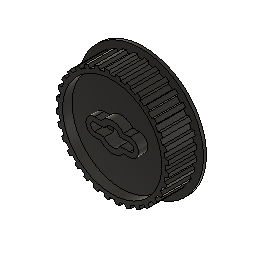
ENGRENAGEM_MEDIA Modificada v1 (Autodesk Fusion 360 design; units mm, degrees)
Autodesk Fusion 360 part; units mm, degrees
note: some values were not read from the file. Set by a fixed rule: which sketch regions a step uses.
sketch "Esboço1" plane through (0, 0, 0) normal (0, 1, 0) x (1, 0, 0)
  circle A0 centre (0, 0) radius 24.25
  line L0 (-0.0462, -30) -> (-0.0462, 30) construction
  circle A1 centre (0, 0) radius 4
  circle A2 centre (0, 0) radius 6.5
  line L1 (0, 0) -> (9.8, 0) construction
  line L2 (0, 0) -> (-9.8, 0) construction
  line L3 (-8, -1.8) -> (8, -1.8)
  arc A3 (8, -1.8) -> (8, 1.8) centre (8, 0) ccw
  line L4 (8, 1.8) -> (-8, 1.8)
  arc A4 (-8, 1.8) -> (-8, -1.8) centre (-8, 0) ccw
  line L5 (-8, 0) -> (8, 0) construction
  line L6 (8, 4) -> (-8, 4)
  arc A5 (-8, 4) -> (-8, -4) centre (-8, 0) ccw
  line L7 (-8, -4) -> (8, -4)
  arc A6 (8, -4) -> (8, 4) centre (8, 0) ccw
  line L8 (8, 0) -> (-8, 0) construction
  circle A7 centre (0, 0) radius 22.561
  circle A8 centre (0, 0) radius 25.6
  line L9 (1.1957, -24.2693) -> (1.7958, -25.976)
  line L10 (-1.0097, -24.2452) -> (1.1957, -24.2693)
  line L11 (1.7958, -25.976) -> (-1.647, -25.9383)
  line L12 (-1.647, -25.9383) -> (-1.0097, -24.2452)
  circle A9 centre (0, 0) radius 25.7968
  line L13 (3.7397, -23.9763) -> (5.9074, -23.5697)
  line L14 (6.829, -25.1265) -> (3.445, -25.7612)
  line L15 (3.445, -25.7612) -> (3.7397, -23.9763)
  line L16 (5.9074, -23.5697) -> (6.829, -25.1265)
  line L17 (8.3454, -22.786) -> (10.3921, -21.9643)
  line L18 (11.5997, -23.3114) -> (8.4045, -24.5941)
  line L19 (8.4045, -24.5941) -> (8.3454, -22.786)
  line L20 (10.3921, -21.9643) -> (11.5997, -23.3114)
  line L21 (12.6304, -20.7201) -> (14.4775, -19.5149)
  line L22 (15.9246, -20.6005) -> (13.0411, -22.4819)
  line L23 (13.0411, -22.4819) -> (12.6304, -20.7201)
  line L24 (14.4775, -19.5149) -> (15.9246, -20.6005)
  line L25 (16.43, -17.8579) -> (18.0065, -16.3155)
  line L26 (19.6376, -17.098) -> (17.1766, -19.5057)
  line L27 (17.1766, -19.5057) -> (16.43, -17.8579)
  line L28 (18.0065, -16.3155) -> (19.6376, -17.098)
  line L29 (19.5982, -14.3094) -> (20.8435, -12.4891)
  line L30 (22.5959, -12.9383) -> (20.6519, -15.78)
  line L31 (20.6519, -15.78) -> (19.5982, -14.3094)
  line L32 (20.8435, -12.4891) -> (22.5959, -12.9383)
  line L33 (22.0132, -10.211) -> (22.8795, -8.1828)
  line L34 (24.6859, -8.2815) -> (23.3336, -11.4478)
  line L35 (23.3336, -11.4478) -> (22.0132, -10.211)
  line L36 (22.8795, -8.1828) -> (24.6859, -8.2815)
  line L37 (23.5823, -5.7203) -> (24.0362, -3.562)
  line L38 (25.8272, -3.3064) -> (25.1186, -6.6756)
  line L39 (25.1186, -6.6756) -> (23.5823, -5.7203)
  line L40 (24.0362, -3.562) -> (25.8272, -3.3064)
  line L41 (24.2452, -1.0097) -> (24.2693, 1.1957)
  line L42 (25.976, 1.7958) -> (25.9383, -1.647)
  line L43 (25.9383, -1.647) -> (24.2452, -1.0097)
  line L44 (24.2693, 1.1957) -> (25.976, 1.7958)
  line L45 (23.9763, 3.7397) -> (23.5697, 5.9074)
  line L46 (25.1265, 6.829) -> (25.7612, 3.445)
  line L47 (25.7612, 3.445) -> (23.9763, 3.7397)
  line L48 (23.5697, 5.9074) -> (25.1265, 6.829)
  line L49 (22.786, 8.3454) -> (21.9643, 10.3921)
  line L50 (23.3114, 11.5997) -> (24.5941, 8.4045)
  line L51 (24.5941, 8.4045) -> (22.786, 8.3454)
  line L52 (21.9643, 10.3921) -> (23.3114, 11.5997)
  line L53 (20.7201, 12.6304) -> (19.5149, 14.4775)
  line L54 (20.6005, 15.9246) -> (22.4819, 13.0411)
  line L55 (22.4819, 13.0411) -> (20.7201, 12.6304)
  line L56 (19.5149, 14.4775) -> (20.6005, 15.9246)
  line L57 (17.8579, 16.43) -> (16.3155, 18.0065)
  line L58 (17.098, 19.6376) -> (19.5057, 17.1766)
  line L59 (19.5057, 17.1766) -> (17.8579, 16.43)
  line L60 (16.3155, 18.0065) -> (17.098, 19.6376)
  line L61 (14.3094, 19.5982) -> (12.4891, 20.8435)
  line L62 (12.9383, 22.5959) -> (15.78, 20.6519)
  line L63 (15.78, 20.6519) -> (14.3094, 19.5982)
  line L64 (12.4891, 20.8435) -> (12.9383, 22.5959)
  line L65 (10.211, 22.0132) -> (8.1828, 22.8795)
  line L66 (8.2815, 24.6859) -> (11.4478, 23.3336)
  line L67 (11.4478, 23.3336) -> (10.211, 22.0132)
  line L68 (8.1828, 22.8795) -> (8.2815, 24.6859)
  line L69 (5.7203, 23.5823) -> (3.562, 24.0362)
  line L70 (3.3064, 25.8272) -> (6.6756, 25.1186)
  line L71 (6.6756, 25.1186) -> (5.7203, 23.5823)
  line L72 (3.562, 24.0362) -> (3.3064, 25.8272)
  line L73 (1.0097, 24.2452) -> (-1.1957, 24.2693)
  line L74 (-1.7958, 25.976) -> (1.647, 25.9383)
  line L75 (1.647, 25.9383) -> (1.0097, 24.2452)
  line L76 (-1.1957, 24.2693) -> (-1.7958, 25.976)
  line L77 (-3.7397, 23.9763) -> (-5.9074, 23.5697)
  line L78 (-6.829, 25.1265) -> (-3.445, 25.7612)
  line L79 (-3.445, 25.7612) -> (-3.7397, 23.9763)
  line L80 (-5.9074, 23.5697) -> (-6.829, 25.1265)
  line L81 (-8.3454, 22.786) -> (-10.3921, 21.9643)
  line L82 (-11.5997, 23.3114) -> (-8.4045, 24.5941)
  line L83 (-8.4045, 24.5941) -> (-8.3454, 22.786)
  line L84 (-10.3921, 21.9643) -> (-11.5997, 23.3114)
  line L85 (-12.6304, 20.7201) -> (-14.4775, 19.5149)
  line L86 (-15.9246, 20.6005) -> (-13.0411, 22.4819)
  line L87 (-13.0411, 22.4819) -> (-12.6304, 20.7201)
  line L88 (-14.4775, 19.5149) -> (-15.9246, 20.6005)
  line L89 (-16.43, 17.8579) -> (-18.0065, 16.3155)
  line L90 (-19.6376, 17.098) -> (-17.1766, 19.5057)
  line L91 (-17.1766, 19.5057) -> (-16.43, 17.8579)
  line L92 (-18.0065, 16.3155) -> (-19.6376, 17.098)
  line L93 (-19.5982, 14.3094) -> (-20.8435, 12.4891)
  line L94 (-22.5959, 12.9383) -> (-20.6519, 15.78)
  line L95 (-20.6519, 15.78) -> (-19.5982, 14.3094)
  line L96 (-20.8435, 12.4891) -> (-22.5959, 12.9383)
  line L97 (-22.0132, 10.211) -> (-22.8795, 8.1828)
  line L98 (-24.6859, 8.2815) -> (-23.3336, 11.4478)
  line L99 (-23.3336, 11.4478) -> (-22.0132, 10.211)
  line L100 (-22.8795, 8.1828) -> (-24.6859, 8.2815)
  line L101 (-23.5823, 5.7203) -> (-24.0362, 3.562)
  line L102 (-25.8272, 3.3064) -> (-25.1186, 6.6756)
  line L103 (-25.1186, 6.6756) -> (-23.5823, 5.7203)
  line L104 (-24.0362, 3.562) -> (-25.8272, 3.3064)
  line L105 (-24.2452, 1.0097) -> (-24.2693, -1.1957)
  line L106 (-25.976, -1.7958) -> (-25.9383, 1.647)
  line L107 (-25.9383, 1.647) -> (-24.2452, 1.0097)
  line L108 (-24.2693, -1.1957) -> (-25.976, -1.7958)
  line L109 (-23.9763, -3.7397) -> (-23.5697, -5.9074)
  line L110 (-25.1265, -6.829) -> (-25.7612, -3.445)
  line L111 (-25.7612, -3.445) -> (-23.9763, -3.7397)
  line L112 (-23.5697, -5.9074) -> (-25.1265, -6.829)
  line L113 (-22.786, -8.3454) -> (-21.9643, -10.3921)
  line L114 (-23.3114, -11.5997) -> (-24.5941, -8.4045)
  line L115 (-24.5941, -8.4045) -> (-22.786, -8.3454)
  line L116 (-21.9643, -10.3921) -> (-23.3114, -11.5997)
  line L117 (-20.7201, -12.6304) -> (-19.5149, -14.4775)
  line L118 (-20.6005, -15.9246) -> (-22.4819, -13.0411)
  line L119 (-22.4819, -13.0411) -> (-20.7201, -12.6304)
  line L120 (-19.5149, -14.4775) -> (-20.6005, -15.9246)
  line L121 (-17.8579, -16.43) -> (-16.3155, -18.0065)
  line L122 (-17.098, -19.6376) -> (-19.5057, -17.1766)
  line L123 (-19.5057, -17.1766) -> (-17.8579, -16.43)
  line L124 (-16.3155, -18.0065) -> (-17.098, -19.6376)
  line L125 (-14.3094, -19.5982) -> (-12.4891, -20.8435)
  line L126 (-12.9383, -22.5959) -> (-15.78, -20.6519)
  line L127 (-15.78, -20.6519) -> (-14.3094, -19.5982)
  line L128 (-12.4891, -20.8435) -> (-12.9383, -22.5959)
  line L129 (-10.211, -22.0132) -> (-8.1828, -22.8795)
  line L130 (-8.2815, -24.6859) -> (-11.4478, -23.3336)
  line L131 (-11.4478, -23.3336) -> (-10.211, -22.0132)
  line L132 (-8.1828, -22.8795) -> (-8.2815, -24.6859)
  line L133 (-5.7203, -23.5823) -> (-3.562, -24.0362)
  line L134 (-3.3064, -25.8272) -> (-6.6756, -25.1186)
  line L135 (-6.6756, -25.1186) -> (-5.7203, -23.5823)
  line L136 (-3.562, -24.0362) -> (-3.3064, -25.8272)
  dimension "d2" = 48.5
  dimension "d7" = 8
  dimension "d8" = 13
  dimension "d10" = 9.8
  dimension "d11" = 9.8
  dimension "d12" = 4
  dimension "d19" = 45.1221
  dimension "d27" = 1.8
  dimension "d65" = 51.2
  dimension "d111" = 70
  dimension "d112" = 70
  dimension "d113" = 2.2055
  dimension "d114" = 3.443
  dimension "d116" = 51.5937
  dimension "d118" = 360
  constraint coincident A0.centre A1.centre
  constraint vertical L0
  constraint concentric A0 A1
  constraint perpendicular L0 L1
  constraint perpendicular L0 L2
  constraint tangent L3 A3
  constraint tangent A3 L4
  constraint parallel L3 L4
  constraint tangent L4 A4
  constraint tangent L3 A4
  constraint coincident L1 A3.centre
  constraint parallel L1 L5
  constraint tangent L6 A5
  constraint tangent A5 L7
  constraint parallel L6 L7
  constraint tangent L7 A6
  constraint tangent L6 A6
  constraint coincident A4.centre L5.start
  constraint parallel L2 L8
  constraint coincident A3.centre L5.end
  constraint concentric A0 A7
  constraint concentric A0 A8
  constraint parallel L10 L11
  constraint concentric A0 A9
  measures "d2" diameter of A0
  measures "d7" diameter of A1
  measures "d8" diameter of A2
  measures "d10" distance of A0.centre L2.end
  measures "d11" distance of A0.centre L1.end
  measures "d12" radius of A5
  measures "d19" diameter of A7
  measures "d27" radius of A4
  measures "d65" diameter of A8
  measures "d111" angle of L11 L12
  measures "d112" angle of L9 L11
  measures "d113" distance of L10.start L9.start
  measures "d114" distance of L9.end L11.end
  measures "d116" diameter of A9
extrude "Extrude20" add sketch "Esboço1" along normal blind 13 contours A0 | A1 A2 L3 L4 | A1 A2 L4 L6 | A1 A2 L3 L7 | A2 L6 | A1 A2 L4 L6 | A2 L3 A3 L4 | A2 L3 A3 L4 L6 L7 A6 | A1 A2 L3 L4 | A1 A2 L3 L7 | A2 L7 | A2 L3 L4 A4 L6 A5 L7 | A2 L3 L4 A4 | A7 | A8 L9 L10 L12 L13 L15 L16 L17 L19 L20 L21 L23 L24 L25 L27 L28 L29 L31 L32 L33 L35 L36 L37 L39 L40 L41 L43 L44 L45 L47 L48 L49 L51 L52 L53 L55 L56 L57 L59 L60 L61 L63 L64 L65 L67 L68 L69 L71 L72 L73 L75 L76 L77 L79 L80 L81 L83 L84 L85 L87 L88 L89 L91 L92 L93 L95 L96 L97 L99 L100 L101 L103 L104 L105 L107 L108 L109 L111 L112 L113 L115 L116 L117 L119 L120 L121 L123 L124 L125 L127 L128 L129 L131 L132 L133 L135 L136 makes body 1
extrude "Extrusão10" cut sketch "Esboço1" along normal blind 5.85 contours A2 L3 A3 L4 | A2 L3 L4 A4 bodies 1
extrude "Extrusão11" cut sketch "Esboço1" along normal blind 4.3 contours A1 A2 L3 L4 | A1 A2 L3 L4 bodies 1
extrude "Extrusão12" cut sketch "Esboço1" along normal blind 4.3 contours A7 bodies 1
sketch "Sketch8" plane through (0, 13, 0) normal (0, 1, 0) x (-1, 0, 0)
  circle A0 centre (0, 0) radius 4
  line L0 (3.562, 24.0362) -> (3.3706, 25.3771)
  arc A1 (3.3706, 25.3771) -> (1.503, 25.5558) centre (0, 0) ccw
  line L1 (1.503, 25.5558) -> (1.0097, 24.2452)
  line L2 (1.0097, 24.2452) -> (-1.1957, 24.2693)
  line L3 (-1.1957, 24.2693) -> (-1.645, 25.5471)
  arc A2 (-1.645, 25.5471) -> (-3.5116, 25.358) centre (0, 0) ccw
  line L4 (-3.5116, 25.358) -> (-3.7397, 23.9763)
  line L5 (-3.7397, 23.9763) -> (-5.9074, 23.5697)
  line L6 (-5.9074, 23.5697) -> (-6.5974, 24.7353)
  arc A3 (-6.5974, 24.7353) -> (-8.3912, 24.1857) centre (0, 0) ccw
  line L7 (-8.3912, 24.1857) -> (-8.3454, 22.786)
  line L8 (-8.3454, 22.786) -> (-10.3921, 21.9643)
  line L9 (-10.3921, 21.9643) -> (-11.2962, 22.9729)
  arc A4 (-11.2962, 22.9729) -> (-12.9483, 22.0839) centre (0, 0) ccw
  line L10 (-12.9483, 22.0839) -> (-12.6304, 20.7201)
  line L11 (-12.6304, 20.7201) -> (-14.4775, 19.5149)
  line L12 (-14.4775, 19.5149) -> (-15.561, 20.3277)
  arc A5 (-15.561, 20.3277) -> (-17.0079, 19.1335) centre (0, 0) ccw
  line L13 (-17.0079, 19.1335) -> (-16.43, 17.8579)
  line L14 (-16.43, 17.8579) -> (-18.0065, 16.3155)
  line L15 (-18.0065, 16.3155) -> (-19.2277, 16.9013)
  arc A6 (-19.2277, 16.9013) -> (-20.4139, 15.4478) centre (0, 0) ccw
  line L16 (-20.4139, 15.4478) -> (-19.5982, 14.3094)
  line L17 (-19.5982, 14.3094) -> (-20.8435, 12.4891)
  line L18 (-20.8435, 12.4891) -> (-22.1555, 12.8254)
  arc A7 (-22.1555, 12.8254) -> (-23.0353, 11.1684) centre (0, 0) ccw
  line L19 (-23.0353, 11.1684) -> (-22.0132, 10.211)
  line L20 (-22.0132, 10.211) -> (-22.8795, 8.1828)
  line L21 (-22.8795, 8.1828) -> (-24.2319, 8.2567)
  arc A8 (-24.2319, 8.2567) -> (-24.7716, 6.4598) centre (0, 0) ccw
  line L22 (-24.7716, 6.4598) -> (-23.5823, 5.7203)
  line L23 (-23.5823, 5.7203) -> (-24.0362, 3.562)
  line L24 (-24.0362, 3.562) -> (-25.3771, 3.3706)
  arc A9 (-25.3771, 3.3706) -> (-25.5558, 1.503) centre (0, 0) ccw
  line L25 (-25.5558, 1.503) -> (-24.2452, 1.0097)
  line L26 (-24.2452, 1.0097) -> (-24.2693, -1.1957)
  line L27 (-24.2693, -1.1957) -> (-25.5471, -1.645)
  arc A10 (-25.5471, -1.645) -> (-25.358, -3.5116) centre (0, 0) ccw
  line L28 (-25.358, -3.5116) -> (-23.9763, -3.7397)
  line L29 (-23.9763, -3.7397) -> (-23.5697, -5.9074)
  line L30 (-23.5697, -5.9074) -> (-24.7353, -6.5974)
  arc A11 (-24.7353, -6.5974) -> (-24.1857, -8.3912) centre (0, 0) ccw
  line L31 (-24.1857, -8.3912) -> (-22.786, -8.3454)
  line L32 (-22.786, -8.3454) -> (-21.9643, -10.3921)
  line L33 (-21.9643, -10.3921) -> (-22.9729, -11.2962)
  arc A12 (-22.9729, -11.2962) -> (-22.0839, -12.9483) centre (0, 0) ccw
  line L34 (-22.0839, -12.9483) -> (-20.7201, -12.6304)
  line L35 (-20.7201, -12.6304) -> (-19.5149, -14.4775)
  line L36 (-19.5149, -14.4775) -> (-20.3277, -15.561)
  arc A13 (-20.3277, -15.561) -> (-19.1335, -17.0079) centre (0, 0) ccw
  line L37 (-19.1335, -17.0079) -> (-17.8579, -16.43)
  line L38 (-17.8579, -16.43) -> (-16.3155, -18.0065)
  line L39 (-16.3155, -18.0065) -> (-16.9013, -19.2277)
  arc A14 (-16.9013, -19.2277) -> (-15.4478, -20.4139) centre (0, 0) ccw
  line L40 (-15.4478, -20.4139) -> (-14.3094, -19.5982)
  line L41 (-14.3094, -19.5982) -> (-12.4891, -20.8435)
  line L42 (-12.4891, -20.8435) -> (-12.8254, -22.1555)
  arc A15 (-12.8254, -22.1555) -> (-11.1684, -23.0353) centre (0, 0) ccw
  line L43 (-11.1684, -23.0353) -> (-10.211, -22.0132)
  line L44 (-10.211, -22.0132) -> (-8.1828, -22.8795)
  line L45 (-8.1828, -22.8795) -> (-8.2567, -24.2319)
  arc A16 (-8.2567, -24.2319) -> (-6.4598, -24.7716) centre (0, 0) ccw
  line L46 (-6.4598, -24.7716) -> (-5.7203, -23.5823)
  line L47 (-5.7203, -23.5823) -> (-3.562, -24.0362)
  line L48 (-3.562, -24.0362) -> (-3.3706, -25.3771)
  arc A17 (-3.3706, -25.3771) -> (-1.503, -25.5558) centre (0, 0) ccw
  line L49 (-1.503, -25.5558) -> (-1.0097, -24.2452)
  line L50 (-1.0097, -24.2452) -> (1.1957, -24.2693)
  line L51 (1.1957, -24.2693) -> (1.645, -25.5471)
  arc A18 (1.645, -25.5471) -> (3.5116, -25.358) centre (0, 0) ccw
  line L52 (3.5116, -25.358) -> (3.7397, -23.9763)
  line L53 (3.7397, -23.9763) -> (5.9074, -23.5697)
  line L54 (5.9074, -23.5697) -> (6.5974, -24.7353)
  arc A19 (6.5974, -24.7353) -> (8.3912, -24.1857) centre (0, 0) ccw
  line L55 (8.3912, -24.1857) -> (8.3454, -22.786)
  line L56 (8.3454, -22.786) -> (10.3921, -21.9643)
  line L57 (10.3921, -21.9643) -> (11.2962, -22.9729)
  arc A20 (11.2962, -22.9729) -> (12.9483, -22.0839) centre (0, 0) ccw
  line L58 (12.9483, -22.0839) -> (12.6304, -20.7201)
  line L59 (12.6304, -20.7201) -> (14.4775, -19.5149)
  line L60 (14.4775, -19.5149) -> (15.561, -20.3277)
  arc A21 (15.561, -20.3277) -> (17.0079, -19.1335) centre (0, 0) ccw
  line L61 (17.0079, -19.1335) -> (16.43, -17.8579)
  line L62 (16.43, -17.8579) -> (18.0065, -16.3155)
  line L63 (18.0065, -16.3155) -> (19.2277, -16.9013)
  arc A22 (19.2277, -16.9013) -> (20.4139, -15.4478) centre (0, 0) ccw
  line L64 (20.4139, -15.4478) -> (19.5982, -14.3094)
  line L65 (19.5982, -14.3094) -> (20.8435, -12.4891)
  line L66 (20.8435, -12.4891) -> (22.1555, -12.8254)
  arc A23 (22.1555, -12.8254) -> (23.0353, -11.1684) centre (0, 0) ccw
  line L67 (23.0353, -11.1684) -> (22.0132, -10.211)
  line L68 (22.0132, -10.211) -> (22.8795, -8.1828)
  line L69 (22.8795, -8.1828) -> (24.2319, -8.2567)
  arc A24 (24.2319, -8.2567) -> (24.7716, -6.4598) centre (0, 0) ccw
  line L70 (24.7716, -6.4598) -> (23.5823, -5.7203)
  line L71 (23.5823, -5.7203) -> (24.0362, -3.562)
  line L72 (24.0362, -3.562) -> (25.3771, -3.3706)
  arc A25 (25.3771, -3.3706) -> (25.5558, -1.503) centre (0, 0) ccw
  line L73 (25.5558, -1.503) -> (24.2452, -1.0097)
  line L74 (24.2452, -1.0097) -> (24.2693, 1.1957)
  line L75 (24.2693, 1.1957) -> (25.5471, 1.645)
  arc A26 (25.5471, 1.645) -> (25.358, 3.5116) centre (0, 0) ccw
  line L76 (25.358, 3.5116) -> (23.9763, 3.7397)
  line L77 (23.9763, 3.7397) -> (23.5697, 5.9074)
  line L78 (23.5697, 5.9074) -> (24.7353, 6.5974)
  arc A27 (24.7353, 6.5974) -> (24.1857, 8.3912) centre (0, 0) ccw
  line L79 (24.1857, 8.3912) -> (22.786, 8.3454)
  line L80 (22.786, 8.3454) -> (21.9643, 10.3921)
  line L81 (21.9643, 10.3921) -> (22.9729, 11.2962)
  arc A28 (22.9729, 11.2962) -> (22.0839, 12.9483) centre (0, 0) ccw
  line L82 (22.0839, 12.9483) -> (20.7201, 12.6304)
  line L83 (20.7201, 12.6304) -> (19.5149, 14.4775)
  line L84 (19.5149, 14.4775) -> (20.3277, 15.561)
  arc A29 (20.3277, 15.561) -> (19.1335, 17.0079) centre (0, 0) ccw
  line L85 (19.1335, 17.0079) -> (17.8579, 16.43)
  line L86 (17.8579, 16.43) -> (16.3155, 18.0065)
  line L87 (16.3155, 18.0065) -> (16.9013, 19.2277)
  arc A30 (16.9013, 19.2277) -> (15.4478, 20.4139) centre (0, 0) ccw
  line L88 (15.4478, 20.4139) -> (14.3094, 19.5982)
  line L89 (14.3094, 19.5982) -> (12.4891, 20.8435)
  line L90 (12.4891, 20.8435) -> (12.8254, 22.1555)
  arc A31 (12.8254, 22.1555) -> (11.1684, 23.0353) centre (0, 0) ccw
  line L91 (11.1684, 23.0353) -> (10.211, 22.0132)
  line L92 (10.211, 22.0132) -> (8.1828, 22.8795)
  line L93 (8.1828, 22.8795) -> (8.2567, 24.2319)
  arc A32 (8.2567, 24.2319) -> (6.4598, 24.7716) centre (0, 0) ccw
  line L94 (6.4598, 24.7716) -> (5.7203, 23.5823)
  line L95 (5.7203, 23.5823) -> (3.562, 24.0362)
  circle A33 centre (0, 0) radius 28.5
  dimension "d123" = 57
  constraint concentric A0 A33
  measures "d123" diameter of A33
extrude "Extrude21" add sketch "Sketch8" along normal blind 1.35 separate body contours L0 A1 L1 L2 L3 A2 L4 L5 L6 A3 L7 L8 L9 A4 L10 L11 L12 A5 L13 L14 L15 A6 L16 L17 L18 A7 L19 L20 L21 A8 L22 L23 L24 A9 L25 L26 L27 A10 L28 L29 L30 A11 L31 L32 L33 A12 L34 L35 L36 A13 L37 L38 L39 A14 L40 L41 L42 A15 L43 L44 L45 A16 L46 L47 L48 A17 L49 L50 L51 A18 L52 L53 L54 A19 L55 L56 L57 A20 L58 L59 L60 A21 L61 L62 L63 A22 L64 L65 L66 A23 L67 L68 L69 A24 L70 L71 L72 A25 L73 L74 L75 A26 L76 L77 L78 A27 L79 L80 L81 A28 L82 L83 L84 A29 L85 L86 L87 A30 L88 L89 L90 A31 L91 L92 L93 A32 L94 L95 | A33 makes body 2
sketch "Esboço7" plane through (0, 14.35, 0) normal (0, 1, 0) x (-1, 0, 0)
  circle A0 centre (0, 0) radius 28.5
  arc A1 (-8, 4.0426) -> (-8, -3.9574) centre (-8, 0.0426) ccw
  arc A2 (8, -3.9574) -> (8, 4.0426) centre (8, 0.0426) ccw
  arc A3 (-8, 1.8426) -> (-8, -1.7574) centre (-8, 0.0426) ccw
  arc A4 (8, -1.7574) -> (8, 1.8426) centre (8, 0.0426) ccw
  line L0 (-8, 4.0426) -> (8, 4.0426)
  line L1 (-8, -3.9574) -> (8, -3.9574)
  line L2 (-8, -1.7574) -> (8, -1.7574)
  line L3 (-8, 1.8426) -> (8, 1.8426)
  circle A5 centre (0, 0) radius 4
  circle A6 centre (0, 0) radius 6.5
  circle A7 centre (0, 0) radius 22.561
  dimension "d98" = 16
  dimension "d100" = 8
  dimension "d101" = 8
  dimension "d102" = 8
  dimension "d103" = 13
  dimension "d104" = 45.122
  constraint concentric A1 A3
  constraint concentric A2 A4
  constraint tangent A2 L0
  constraint tangent A2 L1
  constraint tangent A4 L2
  constraint tangent A4 L3
  constraint concentric A0 A5
  constraint concentric A0 A6
  constraint concentric A5 A7
  measures "d98" distance of A3.start A4.end
  measures "d100" horizontal distance of A2.centre A0.centre
  measures "d101" horizontal distance of A1.centre A0.centre
  measures "d102" diameter of A5
  measures "d103" diameter of A6
  measures "d104" diameter of A7
extrude "Extrude22" cut sketch "Esboço7" against normal blind 4.3 contours A7 bodies 1 2 makes body 3 at (-26.3302, 13, -2.5367)
extrude "Extrude23" cut sketch "Esboço7" against normal blind 5.85 contours A3 L2 L3 A6 | A4 L2 L3 A6 bodies 1 2
extrude "Extrude24" cut sketch "Esboço7" against normal blind 4.3 contours L2 L3 A5 A6 | L2 L3 A5 A6 bodies 1 2
